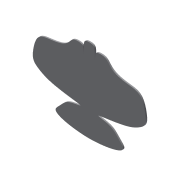
# Autodesk Inventor part: rubberFlatPattern
Saved by Autodesk Inventor 2018 (Build 220112000, 112)
## iProperties
Created: 2020-03-23
Part Number: rubberFlatPattern
Material: Generic
Document SubType Name: Modeling
Designer: Matt
Density: 1 g/cm^3
Appearance: Default
Author: Matt
Autodesk Inventor part; units mm, degrees
ref_plane "YZ Plane" through (0, 0, 0) normal (1, 0, 0) x (0, 1, 0)
ref_plane "XZ Plane" through (0, 0, 0) normal (0, 1, 0) x (-1, 0, 0)
ref_plane "XY Plane" through (0, 0, 0) normal (0, 0, 1) x (1, 0, 0)
sketch "Sketch1" plane through (0, 0, 0) normal (0, 0, 1) x (1, 0, 0)
  line L0 (-8.4915, 78.1346) -> (0.9326, 78.1346) construction
  line L1 (0.9326, 78.1346) -> (1.3054, 70.593) construction
  line L2 (1.3054, 70.593) -> (1.3054, 54.6641) construction
  line L3 (1.3054, 54.6641) -> (1.3054, 52.4045) construction
  line L4 (19.8844, 70.593) -> (24.4248, 64.2345) construction
  line L5 (24.4248, 64.2345) -> (33.721, 51.8234) construction
  line L6 (33.721, 51.8234) -> (59.0059, 47.5048) construction
  line L7 (59.0059, 47.5048) -> (78.354, 46.942) construction
  line L8 (78.354, 46.942) -> (87.4157, 33.9543) construction
  line L9 (87.4157, 33.9543) -> (90.819, 17.0222) construction
  line L10 (90.819, 17.0222) -> (92.9485, 0) construction
  line L11 (92.9485, 0) -> (79.5979, -7.9267) construction
  line L12 (79.5979, -7.9267) -> (62.9837, -17.7912) construction
  line L13 (62.9837, -17.7912) -> (18.0015, -24.0421) construction
  line L14 (18.0015, -24.0421) -> (5.8254, -25.5939) construction
  line L15 (5.8254, -25.5939) -> (5.8254, -27.0264) construction
  line L16 (5.8254, -27.0264) -> (29.0729, -29.9265) construction
  line L17 (29.0729, -29.9265) -> (37.1011, -37.1731) construction
  line L18 (37.1011, -37.1731) -> (45.696, -47.0811) construction
  line L19 (45.696, -47.0811) -> (54.4862, -54.4928) construction
  line L20 (54.4862, -54.4928) -> (46.3634, -61.6031) construction
  line L21 (46.3634, -61.6031) -> (25.7015, -66.9) construction
  line L22 (25.7015, -66.9) -> (2.0055, -69.0457) construction
  line L23 (2.0055, -69.0457) -> (-8.4915, -69.0457) construction
  spline S0 degree 4 poles (-8.4915, 78.1346) (0.9326, 78.1346) (1.3054, 70.593) (1.3054, 54.6641) (1.3054, 52.4045) (1.7957, 65.1079) (3.3868, 69.6522) (19.8844, 70.593) (24.4248, 64.2345) (33.721, 51.8234) (59.0059, 47.5048) (78.354, 46.942) (87.4157, 33.9543) (90.819, 17.0222) (92.9485, 0) (79.5979, -7.9267) (62.9837, -17.7912) (18.0015, -24.0421) (5.8254, -25.5939) (5.8254, -27.0264) (29.0729, -29.9265) (37.1011, -37.1731) (45.696, -47.0811) (54.4862, -54.4928) (46.3634, -61.6031) (25.7015, -66.9) (2.0055, -69.0457) (-8.4915, -69.0457) knots 1 1 1 1 1 2 3 4 4.801491 5 6 7 8 9 10 11 12 13 14 15 16 17 18 19 20 21 22 23 24 24 24 24 24
  line L24 (1.3054, 52.4045) -> (1.7957, 65.1079) construction
  line L25 (1.7957, 65.1079) -> (3.3868, 69.6522) construction
  line L26 (3.3868, 69.6522) -> (19.8844, 70.593) construction
  line L27 (-8.4915, 78.1346) -> (-8.4915, -69.0457)
  line L28 (-8.4915, 78.1346) -> (-17.9156, 78.1346) construction
  line L29 (-17.9156, 78.1346) -> (-18.2885, 70.593) construction
  line L30 (-18.2885, 70.593) -> (-18.2885, 54.6641) construction
  line L31 (-18.2885, 54.6641) -> (-18.2885, 52.4045) construction
  line L32 (-36.8674, 70.593) -> (-41.4079, 64.2345) construction
  line L33 (-41.4079, 64.2345) -> (-50.7041, 51.8234) construction
  line L34 (-50.7041, 51.8234) -> (-75.9889, 47.5048) construction
  line L35 (-75.9889, 47.5048) -> (-95.337, 46.942) construction
  line L36 (-95.337, 46.942) -> (-104.3988, 33.9543) construction
  line L37 (-104.3988, 33.9543) -> (-107.802, 17.0222) construction
  line L38 (-107.802, 17.0222) -> (-109.9316, 0) construction
  line L39 (-109.9316, 0) -> (-96.581, -7.9267) construction
  line L40 (-96.581, -7.9267) -> (-79.9667, -17.7912) construction
  line L41 (-79.9667, -17.7912) -> (-34.9845, -24.0421) construction
  line L42 (-34.9845, -24.0421) -> (-22.8085, -25.5939) construction
  line L43 (-22.8085, -25.5939) -> (-22.8085, -27.0264) construction
  line L44 (-22.8085, -27.0264) -> (-46.056, -29.9265) construction
  line L45 (-46.056, -29.9265) -> (-54.0842, -37.1731) construction
  line L46 (-54.0842, -37.1731) -> (-62.679, -47.0811) construction
  line L47 (-62.679, -47.0811) -> (-71.4693, -54.4928) construction
  line L48 (-71.4693, -54.4928) -> (-63.3465, -61.6031) construction
  line L49 (-63.3465, -61.6031) -> (-42.6846, -66.9) construction
  line L50 (-42.6846, -66.9) -> (-18.9885, -69.0457) construction
  line L51 (-18.9885, -69.0457) -> (-8.4915, -69.0457) construction
  spline S1 degree 4 poles (-8.4915, 78.1346) (-17.9156, 78.1346) (-18.2885, 70.593) (-18.2885, 54.6641) (-18.2885, 52.4045) (-18.7788, 65.1079) (-20.3699, 69.6522) (-36.8674, 70.593) (-41.4079, 64.2345) (-50.7041, 51.8234) (-75.9889, 47.5048) (-95.337, 46.942) (-104.3988, 33.9543) (-107.802, 17.0222) (-109.9316, 0) (-96.581, -7.9267) (-79.9667, -17.7912) (-34.9845, -24.0421) (-22.8085, -25.5939) (-22.8085, -27.0264) (-46.056, -29.9265) (-54.0842, -37.1731) (-62.679, -47.0811) (-71.4693, -54.4928) (-63.3465, -61.6031) (-42.6846, -66.9) (-18.9885, -69.0457) (-8.4915, -69.0457) knots 1 1 1 1 1 2 3 4 4.801491 5 6 7 8 9 10 11 12 13 14 15 16 17 18 19 20 21 22 23 24 24 24 24 24
  line L52 (-18.2885, 52.4045) -> (-18.7788, 65.1079) construction
  line L53 (-18.7788, 65.1079) -> (-20.3699, 69.6522) construction
  line L54 (-20.3699, 69.6522) -> (-36.8674, 70.593) construction
  point P0 (0, 0)
  constraints: 26 symmetric about line, 2 end point, 2 vertical, 1 horizontal, 1 perpendicular, 6 other
extrude "Extrusion1" add sketch "Sketch1" along normal blind 2.3813
body "Solid1"
